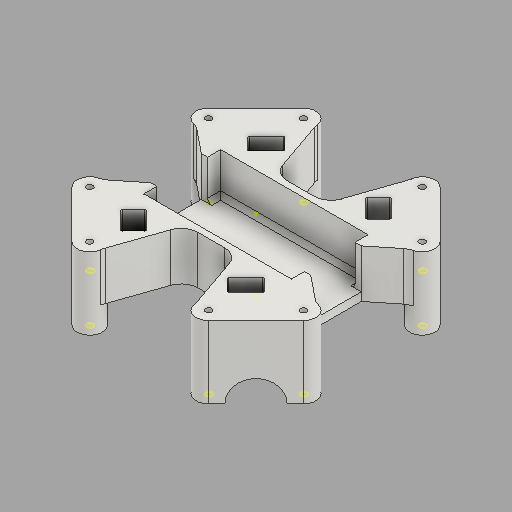
# Autodesk Inventor part: motor_converter
Saved by Autodesk Inventor 2023 (Build 270158000, 158)
## iProperties
Created: 2024-10-30
Part Number: motor_converter
Material: Полиэтилен, низкая плотность
Document SubType Name: Modeling
Designer: Ivan
Density: 0.894 g/cm^3
Appearance: Сталь
Mass: 114.342 g
Surface Area: 371.209 cm^2
Volume: 127.899 cm^3
Author: Ivan
Autodesk Inventor part; units mm, degrees
ref_plane "YZ Plane" through (0, 0, 0) normal (1, 0, 0) x (0, 1, 0)
ref_plane "XZ Plane" through (0, 0, 0) normal (0, 1, 0) x (-1, 0, 0)
ref_plane "XY Plane" through (0, 0, 0) normal (0, 0, 1) x (1, 0, 0)
derived "floor_v2.ipt"
sketch "Эскиз3" plane through (0, 2, 0) normal (0, -1, 0) x (-1, 0, 0)
  line L0 (33.8509, 77.6915) -> (77.6915, 33.8509) construction
  line L1 (55.7712, 55.7712) -> (0, 0) construction
  line L2 (44.4575, 67.0849) -> (67.0849, 44.4575) construction
  circle A0 centre (44.4575, 67.0849) radius 1.5
  circle A1 centre (67.0849, 44.4575) radius 1.5
  line L3 (28.3991, 51.0265) -> (51.0265, 28.3991) construction
  circle A2 centre (28.3991, 51.0265) radius 1.5
  circle A3 centre (51.0265, 28.3991) radius 1.5
  line L4 (44.4575, -67.0849) -> (67.0849, -44.4575) construction
  line L5 (28.3991, -51.0265) -> (51.0265, -28.3991) construction
  line L6 (55.7712, -55.7712) -> (0, 0) construction
  line L7 (-55.7712, -55.7712) -> (0, 0) construction
  line L8 (-28.3991, -51.0265) -> (-51.0265, -28.3991) construction
  line L9 (-44.4575, -67.0849) -> (-67.0849, -44.4575) construction
  line L10 (-55.7712, 55.7712) -> (0, 0) construction
  line L11 (-51.0265, 28.3991) -> (-28.3991, 51.0265) construction
  line L12 (-67.0849, 44.4575) -> (-44.4575, 67.0849) construction
  circle A4 centre (-44.4575, 67.0849) radius 1.5
  circle A5 centre (-67.0849, 44.4575) radius 1.5
  circle A6 centre (-28.3991, 51.0265) radius 1.5
  circle A7 centre (-51.0265, 28.3991) radius 1.5
  circle A8 centre (-44.4575, -67.0849) radius 1.5
  circle A9 centre (-67.0849, -44.4575) radius 1.5
  circle A10 centre (-51.0265, -28.3991) radius 1.5
  circle A11 centre (-28.3991, -51.0265) radius 1.5
  circle A12 centre (44.4575, -67.0849) radius 1.5
  circle A13 centre (28.3991, -51.0265) radius 1.5
  circle A14 centre (51.0265, -28.3991) radius 1.5
  circle A15 centre (67.0849, -44.4575) radius 1.5
  line L13 (-38.4471, -82.2877) -> (-82.2877, -38.4471)
  line L14 (82.2877, -38.4471) -> (38.4471, -82.2877)
  line L15 (38.4471, 82.2877) -> (82.2877, 38.4471)
  line L16 (-82.2877, 38.4471) -> (-38.4471, 82.2877)
  line L17 (82.2877, 38.4471) -> (92.1165, 48.2758)
  point P0 (39.7128, 39.7128)
  point P1 (-39.7128, -39.7128)
  point P2 (39.7128, -39.7128)
  point P3 (-39.7128, 39.7128)
  point P4 (-40.1306, -40.1306)
sketch "Эскиз6" plane through (0, 0, 0) normal (0, 1, 0) x (-1, 0, 0)
  circle A0 centre (28.3991, 51.0265) radius 1.5 projected
  circle A1 centre (51.0265, 28.3991) radius 1.5 projected
  line L0 (28.3991, -51.0265) -> (51.0265, -28.3991) construction
  circle A2 centre (28.3991, -51.0265) radius 1.5 projected
  circle A3 centre (-28.3991, -51.0265) radius 1.5 projected
  circle A4 centre (-51.0265, -28.3991) radius 1.5 projected
  circle A5 centre (-51.0265, 28.3991) radius 1.5 projected
  circle A6 centre (-28.3991, 51.0265) radius 1.5 projected
  circle A7 centre (51.0265, 28.3991) radius 6
  circle A8 centre (28.3991, 51.0265) radius 6
  circle A9 centre (51.0265, -28.3991) radius 6
  circle A10 centre (28.3991, -51.0265) radius 6
  circle A11 centre (-28.3991, -51.0265) radius 6
  circle A12 centre (-51.0265, -28.3991) radius 6
  circle A13 centre (-51.0265, 28.3991) radius 6
  circle A14 centre (-28.3991, 51.0265) radius 6
  line L1 (55.2691, 32.6417) -> (46.7838, 24.1564) construction
  line L2 (28.3991, 51.0265) -> (51.0265, 28.3991) construction
  line L3 (32.6417, 55.2691) -> (24.1564, 46.7838) construction
  line L4 (-28.3991, 51.0265) -> (-51.0265, 28.3991) construction
  line L5 (-51.0265, -28.3991) -> (-28.3991, -51.0265) construction
  line L6 (-32.6417, 55.2691) -> (-24.1564, 46.7838) construction
  line L7 (-55.2691, 32.6417) -> (-46.7838, 24.1564) construction
  line L8 (-46.7838, -24.1564) -> (-55.2691, -32.6417) construction
  line L9 (-24.1564, -46.7838) -> (-32.6417, -55.2691) construction
  line L10 (24.1564, -46.7838) -> (32.6417, -55.2691) construction
  line L11 (46.7838, -24.1564) -> (55.2691, -32.6417) construction
  line L12 (32.6417, 55.2691) -> (55.2691, 32.6417)
  line L13 (46.7838, 24.1564) -> (24.1564, 46.7838)
  line L14 (55.2691, -32.6417) -> (32.6417, -55.2691)
  line L15 (24.1564, -46.7838) -> (46.7838, -24.1564)
  line L16 (-24.1564, -46.7838) -> (-46.7838, -24.1564)
  line L17 (-55.2691, -32.6417) -> (-32.6417, -55.2691)
  line L18 (-24.1564, 46.7838) -> (-46.7838, 24.1564)
  line L19 (-55.2691, 32.6417) -> (-32.6417, 55.2691)
  circle A15 centre (51.0265, -28.3991) radius 1.5 projected
  point P0 (0, 0)
  point P1 (-32.6417, -55.2691)
  dimension "d19" = 12
  constraints: 32 end point, 16 point on circle, 15 coincident, 11 perpendicular, 8 midpoint, 7 centre point, 6 equal radius, 4 parallel, 3 tangent, 1 point on line, 4 other
  measures "d19" diameter of A7
extrude "Выдавливание2" add sketch "Эскиз6" against normal blind 34.5 contours A0 | A1 | A2 | A3 | A4 | A5 | A6 | A7 | A7 L13 A8 L12 | A8 | A9 | A9 L14 A10 L15 | A10 | A11 | A11 L17 A12 L16 | A12 | A13 | A13 L19 A14 L18 | A14 | A15
sketch "Эскиз7" plane through (32.6417, -34.5, 55.2691) normal (0.7071068, 0, 0.7071068) x (0.7071068, 0, -0.7071068)
  line L0 (32, 0) -> (0, 0) projected
  line L1 (32, 0) -> (0, 0) projected
  circle A0 centre (16, 0) radius 10.5
  point P0 (16, 34.5)
  point P1 (5.5, 0)
  point P2 (26.5, 0)
  dimension "d23" = 21
  constraints: 1 centre point, 1 midpoint
  measures "d23" diameter of A0
extrude "Выдавливание3" cut sketch "Эскиз7" against normal through all contours L0 A0 picked at (17.9882, 2.8804)
mirror "Зеркальное отражение1" about plane through (0, 0, 0) normal (0, 0, 1) of "Выдавливание3"
sketch "Эскиз8" plane through (0, 0, 0) normal (0, 1, 0) x (1, 0, 0)
  point P0 (0, 0)
sketch "Эскиз9" plane through (0, -34.5, 0) normal (0, -1, 0) x (1, 0, 0)
  circle A0 centre (-28.3991, 51.0265) radius 1.5 projected
  circle A1 centre (-51.0265, 28.3991) radius 1.5 projected
  circle A2 centre (28.3991, 51.0265) radius 1.5 projected
  circle A3 centre (51.0265, 28.3991) radius 1.5 projected
  circle A4 centre (51.0265, -28.3991) radius 1.5 projected
  circle A5 centre (28.3991, -51.0265) radius 1.5 projected
  circle A6 centre (-28.3991, -51.0265) radius 1.5 projected
  circle A7 centre (-51.0265, -28.3991) radius 1.5 projected
  point P0 (0, 0)
extrude "Выдавливание4" cut sketch "Эскиз3" along normal blind 9 contours A2 | A3 | A6 | A7 | A10 | A11 | A13 | A14
extrude "Выдавливание5" cut sketch "Эскиз9" against normal blind 7
sketch "Эскиз10" plane through (0, 0, 0) normal (0, 1, 0) x (1, 0, 0)
  line L0 (-35.225, -18.325) -> (-35.225, 18.325)
  line L1 (-35.225, 18.325) -> (35.225, 18.325)
  line L2 (35.225, 18.325) -> (35.225, -18.325)
  line L3 (35.225, -18.325) -> (-35.225, -18.325)
  circle A0 centre (-51.0265, 28.3991) radius 1.5 projected
  circle A1 centre (-51.0265, -28.3991) radius 1.5 projected
  circle A2 centre (-51.0265, 28.3991) radius 1.5 projected
  line L4 (-51.0265, 28.3991) -> (-51.0265, -28.3991) construction
  line L5 (-35.225, 18.325) -> (35.225, -18.325) construction
  line L6 (-38.225, 21.325) -> (38.225, 21.325)
  line L7 (38.225, 21.325) -> (38.225, -21.325)
  line L8 (38.225, -21.325) -> (-38.225, -21.325)
  line L9 (-38.225, -21.325) -> (-38.225, 21.325)
  line L10 (-38.225, 21.325) -> (38.225, -21.325) construction
  line L11 (-31, 15.1) -> (31, 15.1) construction
  line L12 (0, 0) -> (0, 15.1) construction
  circle A3 centre (-31, 15.1) radius 1.65
  circle A4 centre (31, 15.1) radius 1.65
  line L13 (-35.225, 0) -> (35.225, 0) construction
  circle A5 centre (-31, -15.1) radius 1.65
  circle A6 centre (31, -15.1) radius 1.65
  line L14 (-38.225, 12.1) -> (-35.225, 12.1)
  line L15 (-38.225, -12.1) -> (-35.225, -12.1)
  line L16 (38.225, 12.1) -> (35.225, 12.1)
  line L17 (38.225, -12.1) -> (35.225, -12.1)
  arc A7 (-24.1564, 46.7838) -> (-32.6417, 55.2691) centre (-28.3991, 51.0265) ccw projected
  arc A8 (-55.2691, 32.6417) -> (-46.7838, 24.1564) centre (-51.0265, 28.3991) ccw projected
  arc A9 (-46.7838, -24.1564) -> (-55.2691, -32.6417) centre (-51.0265, -28.3991) ccw projected
  arc A10 (-32.6417, -55.2691) -> (-24.1564, -46.7838) centre (-28.3991, -51.0265) ccw projected
  arc A11 (24.1564, -46.7838) -> (32.6417, -55.2691) centre (28.3991, -51.0265) ccw projected
  arc A12 (55.2691, -32.6417) -> (46.7838, -24.1564) centre (51.0265, -28.3991) ccw projected
  arc A13 (46.7838, 24.1564) -> (55.2691, 32.6417) centre (51.0265, 28.3991) ccw projected
  arc A14 (32.6417, 55.2691) -> (24.1564, 46.7838) centre (28.3991, 51.0265) ccw projected
  circle A15 centre (-28.3991, 51.0265) radius 1.5 projected
  line L18 (-28.3991, 51.0265) -> (-24.1564, 55.2691) construction
  line L19 (-28.3991, 51.0265) -> (-24.1564, 46.7838) construction
  arc A16 (-24.1564, 46.7838) -> (-32.6417, 55.2691) centre (-28.3991, 51.0265) ccw projected
  line L20 (-24.1564, 55.2691) -> (-24.1564, 46.7838) construction
  line L21 (-28.3991, 51.0265) -> (-22.3991, 51.0265)
  arc A17 (-22.3991, 51.0265) -> (0, 21.325) centre (3.3903, 47.1785) ccw
  arc A18 (-55.2691, 24.1564) -> (-38.225, 12.1) centre (-33.0894, 37.436) ccw
  line L22 (-46.7838, 24.1564) -> (-24.1564, 46.7838) projected
  point P0 (-24.1564, 51.0265)
  dimension "d31" = 70.45
  dimension "d32" = 36.65
  dimension "d33" = 76.45
  dimension "d34" = 42.65
  dimension "d35" = 3.225
  dimension "d36" = 4.225
  dimension "d37" = 3.3
  dimension "d38" = 3
  constraints: 44 end point, 8 point on circle, 8 symmetric about line, 7 midpoint, 6 centre point, 5 perpendicular, 4 parallel, 3 coincident, 3 point on line, 3 vertical, 2 horizontal, 1 equal radius, 2 other
  measures "d31" distance of L0.end L1.end
  measures "d32" distance of L1.end L2.end
  measures "d33" distance of L6.start L6.end
  measures "d34" distance of L6.end L7.end
  measures "d35" distance from line of L1 L12.end
  measures "d36" distance from line of L0 L11.start
  measures "d37" diameter of A3
  measures "d38" distance from line of L11 L14.end
extrude "Выдавливание6" add sketch "Эскиз10" against normal blind 17 contours L3 L2 L17 L7 L8 L9 L15 L0 | L14 L9 L6 L7 L16 L2 L1 L0
sketch "Эскиз11" plane through (0, -17, 0) normal (0, -1, 0) x (1, 0, 0)
  line L0 (-38.225, 21.325) -> (-38.225, 12.1) projected
  line L1 (-38.225, -21.325) -> (38.225, -21.325) projected
  line L2 (-38.225, 21.325) -> (38.225, 21.325)
  line L3 (38.225, 21.325) -> (38.225, -21.325)
  line L4 (38.225, -21.325) -> (-38.225, -21.325)
  line L5 (-38.225, -21.325) -> (-38.225, 21.325)
  circle A0 centre (-31, 15.1) radius 1.65 projected
  circle A1 centre (31, 15.1) radius 1.65 projected
  circle A2 centre (31, -15.1) radius 1.65 projected
  circle A3 centre (-31, -15.1) radius 1.65 projected
  point P0 (0, 0)
  constraints: 8 end point, 2 parallel, 1 horizontal, 1 perpendicular
extrude "Выдавливание7" add sketch "Эскиз11" along normal blind 5 contours L2 L3 L1 L5 L0 | A0 | A1 | A2 | A3
sketch "Эскиз12" plane through (0, 0, 0) normal (0, 1, 0) x (1, 0, 0)
  circle A0 centre (-51.0265, 28.3991) radius 1.5 projected
  circle A1 centre (-28.3991, 51.0265) radius 1.5 projected
  line L0 (-32.6417, 55.2691) -> (-55.2691, 32.6417) projected
  arc A2 (-55.2691, 32.6417) -> (-46.7838, 24.1564) centre (-51.0265, 28.3991) ccw projected
  line L1 (-46.7838, 24.1564) -> (-24.1564, 46.7838) projected
  arc A3 (-24.1564, 46.7838) -> (-32.6417, 55.2691) centre (-28.3991, 51.0265) ccw projected
  circle A4 centre (28.3991, 51.0265) radius 1.5 projected
  circle A5 centre (-28.3991, 51.0265) radius 1.5 projected
  line L2 (28.3991, 51.0265) -> (-28.3991, 51.0265) construction
  circle A6 centre (-51.0265, -28.3991) radius 1.5 projected
  line L3 (-51.0265, 28.3991) -> (-51.0265, -28.3991) construction
  arc A7 (-24.1564, 46.7838) -> (-32.6417, 55.2691) centre (-28.3991, 51.0265) ccw projected
  line L4 (38.225, 21.325) -> (-38.225, 21.325) projected
  line L5 (-38.225, 21.325) -> (-38.225, 12.1) projected
  arc A8 (-55.2691, 32.6417) -> (-46.7838, 24.1564) centre (-51.0265, 28.3991) ccw projected
  line L6 (-51.0265, 22.3991) -> (-38.225, 12.1)
  arc A9 (-24.1564, 46.7838) -> (-32.6417, 55.2691) centre (-28.3991, 51.0265) ccw projected
  line L7 (-22.3991, 51.0265) -> (-12.1, 21.325)
  arc A10 (32.6417, 55.2691) -> (24.1564, 46.7838) centre (28.3991, 51.0265) ccw projected
  line L8 (22.3991, 51.0265) -> (12.1, 21.325)
  arc A11 (46.7838, 24.1564) -> (55.2691, 32.6417) centre (51.0265, 28.3991) ccw projected
  circle A12 centre (51.0265, -28.3991) radius 1.5 projected
  line L9 (51.0265, 28.3991) -> (51.0265, -28.3991) construction
  circle A13 centre (28.3991, -51.0265) radius 1.5 projected
  circle A14 centre (-28.3991, -51.0265) radius 1.5 projected
  line L10 (28.3991, -51.0265) -> (-28.3991, -51.0265) construction
  line L11 (35.225, 12.1) -> (38.225, 12.1) projected
  line L12 (38.225, 12.1) -> (51.0265, 22.3991)
  line L13 (38.225, 12.1) -> (38.225, -12.1) projected
  line L14 (38.225, -12.1) -> (51.0265, -22.3991)
  arc A15 (55.2691, -32.6417) -> (46.7838, -24.1564) centre (51.0265, -28.3991) ccw projected
  arc A16 (24.1564, -46.7838) -> (32.6417, -55.2691) centre (28.3991, -51.0265) ccw projected
  line L15 (22.3991, -51.0265) -> (12.1, -21.325)
  line L16 (38.225, -21.325) -> (-38.225, -21.325) projected
  arc A17 (-32.6417, -55.2691) -> (-24.1564, -46.7838) centre (-28.3991, -51.0265) ccw projected
  line L17 (-38.225, -21.325) -> (38.225, -21.325) projected
  line L18 (-22.3991, -51.0265) -> (-12.1, -21.325)
  line L19 (-38.225, -12.1) -> (-38.225, -21.325) projected
  line L20 (-38.225, -12.1) -> (-51.0265, -22.3991)
  arc A18 (-46.7838, -24.1564) -> (-55.2691, -32.6417) centre (-51.0265, -28.3991) ccw projected
  circle A19 centre (28.3991, 51.0265) radius 1.5 projected
  circle A20 centre (51.0265, 28.3991) radius 1.5 projected
  arc A21 (46.7838, 24.1564) -> (55.2691, 32.6417) centre (51.0265, 28.3991) ccw projected
  line L21 (55.2691, 32.6417) -> (32.6417, 55.2691) projected
  arc A22 (32.6417, 55.2691) -> (24.1564, 46.7838) centre (28.3991, 51.0265) ccw projected
  line L22 (24.1564, 46.7838) -> (46.7838, 24.1564) projected
  circle A23 centre (28.3991, -51.0265) radius 1.5 projected
  circle A24 centre (51.0265, -28.3991) radius 1.5 projected
  line L23 (46.7838, -24.1564) -> (24.1564, -46.7838) projected
  arc A25 (24.1564, -46.7838) -> (32.6417, -55.2691) centre (28.3991, -51.0265) ccw projected
  line L24 (32.6417, -55.2691) -> (55.2691, -32.6417) projected
  arc A26 (55.2691, -32.6417) -> (46.7838, -24.1564) centre (51.0265, -28.3991) ccw projected
  circle A27 centre (-28.3991, -51.0265) radius 1.5 projected
  circle A28 centre (-51.0265, -28.3991) radius 1.5 projected
  line L25 (-24.1564, -46.7838) -> (-46.7838, -24.1564) projected
  arc A29 (-46.7838, -24.1564) -> (-55.2691, -32.6417) centre (-51.0265, -28.3991) ccw projected
  line L26 (-55.2691, -32.6417) -> (-32.6417, -55.2691) projected
  arc A30 (-32.6417, -55.2691) -> (-24.1564, -46.7838) centre (-28.3991, -51.0265) ccw projected
  line L27 (38.225, 12.1) -> (38.225, 21.325) projected
  line L28 (38.225, -21.325) -> (38.225, -12.1) projected
  line L29 (-19.3804, 33.1638) -> (-25.3908, 39.1742)
  line L30 (-25.3908, 39.1742) -> (-34.2296, 30.3354)
  line L31 (-34.2296, 30.3354) -> (-28.2192, 24.325)
  line L32 (-28.2192, 24.325) -> (-19.3804, 33.1638)
  line L33 (0, 51.0265) -> (0, -51.0265) construction
  line L34 (19.3804, 33.1638) -> (25.3908, 39.1742)
  line L35 (25.3908, 39.1742) -> (34.2296, 30.3354)
  line L36 (34.2296, 30.3354) -> (28.2192, 24.325)
  line L37 (28.2192, 24.325) -> (19.3804, 33.1638)
  line L38 (51.0265, 0) -> (-51.0265, 0) construction
  line L39 (-19.3804, -33.1638) -> (-25.3908, -39.1742)
  line L40 (-25.3908, -39.1742) -> (-34.2296, -30.3354)
  line L41 (-34.2296, -30.3354) -> (-28.2192, -24.325)
  line L42 (-28.2192, -24.325) -> (-19.3804, -33.1638)
  line L43 (28.2192, -24.325) -> (19.3804, -33.1638)
  line L44 (19.3804, -33.1638) -> (25.3908, -39.1742)
  line L45 (25.3908, -39.1742) -> (34.2296, -30.3354)
  line L46 (34.2296, -30.3354) -> (28.2192, -24.325)
  point P0 (0, 0)
  point P1 (0, 21.325)
  point P2 (-46.7838, -24.1564)
  point P3 (-24.1564, -46.7838)
  point P4 (46.7838, 24.1564)
  point P5 (24.1564, 46.7838)
  point P6 (46.7838, -24.1564)
  dimension "d47" = 12.1
  dimension "d50" = 3
  dimension "d51" = 3
  dimension "d52" = 8.5
  dimension "d53" = 12.5
  constraints: 60 end point, 12 point on line, 12 symmetric about line, 8 point on circle, 5 midpoint, 3 equal length, 3 parallel, 3 vertical, 2 horizontal, 1 perpendicular
  measures "d47" distance of L7.end point (0, 21.325)
  measures "d50" distance from line of L4 L31.end
  measures "d51" distance from line of L7 L29.start
  measures "d52" distance from line of L32 L29.end
  measures "d53" distance from line of L31 L29.end
extrude "Выдавливание10" add sketch "Эскиз12" against normal up to surface (22 mm away) contours L7 L4 L5 L6 A2 L1 A3 | L4 L8 A10 L22 A11 L12 L27 | L14 A15 L23 A16 L15 L16 L28 | L18 A17 L25 A18 L20 L19 L16
fillet "Сопряжение1" radius 0.5 16 edges at (34.2296, -11, -30.3354) (28.2192, -11, -24.325) (19.3804, -11, -33.1638) (25.3908, -11, -39.1742) (-34.2296, -11, -30.3354) (-28.2192, -11, -24.325) (-19.3804, -11, -33.1638) (-25.3908, -11, -39.1742) (-25.3908, -11, 39.1742) (-19.3804, -11, 33.1638) (-34.2296, -11, 30.3354) (-28.2192, -11, 24.325) (25.3908, -11, 39.1742) (34.2296, -11, 30.3354) (19.3804, -11, 33.1638) (28.2192, -11, 24.325)
fillet "Сопряжение2" radius 8 12 edges at (22.3991, -11, -51.0265) (51.0265, -11, -22.3991) (51.0265, -11, 22.3991) (22.3991, -11, 51.0265) (-51.0265, -11, 22.3991) (-22.3991, -11, 51.0265) (-51.0265, -11, -22.3991) (-22.3991, -11, -51.0265) (12.1, -11, 21.325) (-12.1, -11, 21.325) (12.1, -11, -21.325) (-12.1, -11, -21.325)
sketch "Эскиз13" plane through (0, -22, 0) normal (0, -1, 0) x (1, 0, 0)
  line L0 (-33.8761, 29.9819) -> (-28.5728, 24.6786) projected
  arc A0 (-33.8761, 30.689) -> (-33.8761, 29.9819) centre (-33.5225, 30.3354) ccw projected
  line L1 (-25.7443, 38.8207) -> (-33.8761, 30.689) projected
  arc A1 (-25.0372, 38.8207) -> (-25.7443, 38.8207) centre (-25.3908, 38.4671) ccw projected
  line L2 (-19.7339, 33.5174) -> (-25.0372, 38.8207) projected
  arc A2 (-19.7339, 32.8103) -> (-19.7339, 33.5174) centre (-20.0875, 33.1638) ccw projected
  line L3 (-27.8657, 24.6786) -> (-19.7339, 32.8103) projected
  arc A3 (-28.5728, 24.6786) -> (-27.8657, 24.6786) centre (-28.2192, 25.0321) ccw projected
  line L4 (19.7339, -33.5174) -> (25.0372, -38.8207) projected
  arc A4 (19.7339, -32.8103) -> (19.7339, -33.5174) centre (20.0875, -33.1638) ccw projected
  line L5 (27.8657, -24.6786) -> (19.7339, -32.8103) projected
  arc A5 (28.5728, -24.6786) -> (27.8657, -24.6786) centre (28.2192, -25.0321) ccw projected
  line L6 (33.8761, -29.9819) -> (28.5728, -24.6786) projected
  arc A6 (33.8761, -30.689) -> (33.8761, -29.9819) centre (33.5225, -30.3354) ccw projected
  line L7 (25.7443, -38.8207) -> (33.8761, -30.689) projected
  arc A7 (25.0372, -38.8207) -> (25.7443, -38.8207) centre (25.3908, -38.4671) ccw projected
  line L8 (-33.8761, -30.689) -> (-25.7443, -38.8207) projected
  arc A8 (-33.8761, -29.9819) -> (-33.8761, -30.689) centre (-33.5225, -30.3354) ccw projected
  line L9 (-28.5728, -24.6786) -> (-33.8761, -29.9819) projected
  arc A9 (-27.8657, -24.6786) -> (-28.5728, -24.6786) centre (-28.2192, -25.0321) ccw projected
  line L10 (-19.7339, -32.8103) -> (-27.8657, -24.6786) projected
  arc A10 (-19.7339, -33.5174) -> (-19.7339, -32.8103) centre (-20.0875, -33.1638) ccw projected
  line L11 (-25.0372, -38.8207) -> (-19.7339, -33.5174) projected
  arc A11 (-25.7443, -38.8207) -> (-25.0372, -38.8207) centre (-25.3908, -38.4671) ccw projected
  line L12 (25.0372, 38.8207) -> (19.7339, 33.5174) projected
  arc A12 (25.7443, 38.8207) -> (25.0372, 38.8207) centre (25.3908, 38.4671) ccw projected
  line L13 (33.8761, 30.689) -> (25.7443, 38.8207) projected
  arc A13 (33.8761, 29.9819) -> (33.8761, 30.689) centre (33.5225, 30.3354) ccw projected
  line L14 (28.5728, 24.6786) -> (33.8761, 29.9819) projected
  arc A14 (27.8657, 24.6786) -> (28.5728, 24.6786) centre (28.2192, 25.0321) ccw projected
  line L15 (19.7339, 32.8103) -> (27.8657, 24.6786) projected
  arc A15 (19.7339, 33.5174) -> (19.7339, 32.8103) centre (20.0875, 33.1638) ccw projected
  line L16 (-38.225, 12.1) -> (-38.225, -12.1) projected
  line L17 (-49.3246, -21.0299) -> (-38.225, -12.1) projected
  arc A16 (-52.4463, -22.5695) -> (-49.3246, -21.0299) centre (-54.3393, -14.7967) ccw projected
  arc A17 (-46.7838, -24.1564) -> (-52.4463, -22.5695) centre (-51.0265, -28.3991) ccw projected
  line L18 (-24.1564, -46.7838) -> (-46.7838, -24.1564) projected
  arc A18 (-22.4393, -51.72) -> (-24.1564, -46.7838) centre (-28.3991, -51.0265) ccw projected
  arc A19 (-22.0514, -50.0239) -> (-22.4393, -51.72) centre (-14.4929, -52.6448) ccw projected
  line L19 (-13.9652, -26.7041) -> (-22.0514, -50.0239) projected
  arc A20 (-6.4067, -21.325) -> (-13.9652, -26.7041) centre (-6.4067, -29.325) ccw projected
  line L20 (-6.4067, -21.325) -> (6.4067, -21.325) projected
  arc A21 (13.9652, -26.7041) -> (6.4067, -21.325) centre (6.4067, -29.325) ccw projected
  line L21 (22.0514, -50.0239) -> (13.9652, -26.7041) projected
  arc A22 (22.4393, -51.72) -> (22.0514, -50.0239) centre (14.4929, -52.6448) ccw projected
  arc A23 (24.1564, -46.7838) -> (22.4393, -51.72) centre (28.3991, -51.0265) ccw projected
  line L22 (46.7838, -24.1564) -> (24.1564, -46.7838) projected
  arc A24 (52.4463, -22.5695) -> (46.7838, -24.1564) centre (51.0265, -28.3991) ccw projected
  arc A25 (49.3246, -21.0299) -> (52.4463, -22.5695) centre (54.3393, -14.7967) ccw projected
  line L23 (38.225, -12.1) -> (49.3246, -21.0299) projected
  line L24 (38.225, -12.1) -> (38.225, 12.1) projected
  line L25 (49.3246, 21.0299) -> (38.225, 12.1) projected
  arc A26 (52.4463, 22.5695) -> (49.3246, 21.0299) centre (54.3393, 14.7967) ccw projected
  arc A27 (46.7838, 24.1564) -> (52.4463, 22.5695) centre (51.0265, 28.3991) ccw projected
  line L26 (24.1564, 46.7838) -> (46.7838, 24.1564) projected
  arc A28 (22.4393, 51.72) -> (24.1564, 46.7838) centre (28.3991, 51.0265) ccw projected
  arc A29 (22.0514, 50.0239) -> (22.4393, 51.72) centre (14.4929, 52.6448) ccw projected
  line L27 (13.9652, 26.7041) -> (22.0514, 50.0239) projected
  arc A30 (6.4067, 21.325) -> (13.9652, 26.7041) centre (6.4067, 29.325) ccw projected
  line L28 (6.4067, 21.325) -> (-6.4067, 21.325) projected
  arc A31 (-13.9652, 26.7041) -> (-6.4067, 21.325) centre (-6.4067, 29.325) ccw projected
  line L29 (-22.0514, 50.0239) -> (-13.9652, 26.7041) projected
  arc A32 (-22.4393, 51.72) -> (-22.0514, 50.0239) centre (-14.4929, 52.6448) ccw projected
  arc A33 (-24.1564, 46.7838) -> (-22.4393, 51.72) centre (-28.3991, 51.0265) ccw projected
  line L30 (-46.7838, 24.1564) -> (-24.1564, 46.7838) projected
  arc A34 (-52.4463, 22.5695) -> (-46.7838, 24.1564) centre (-51.0265, 28.3991) ccw projected
  arc A35 (-49.3246, 21.0299) -> (-52.4463, 22.5695) centre (-54.3393, 14.7967) ccw projected
  line L31 (-38.225, 12.1) -> (-49.3246, 21.0299) projected
  point P0 (0, 0)
extrude "Выдавливание11" add sketch "Эскиз13" along normal blind 1
sketch "Эскиз14" plane through (0, -17, 0) normal (0, 1, 0) x (1, 0, 0)
  line L0 (-35.225, 12.1) -> (-38.225, 12.1) projected
  line L1 (-38.225, -12.1) -> (-38.225, 12.1) projected
  line L2 (-38.225, -12.1) -> (-35.225, -12.1) projected
  line L3 (-35.225, -12.1) -> (-35.225, -18.325) projected
  line L4 (-35.225, -18.325) -> (35.225, -18.325) projected
  line L5 (35.225, -18.325) -> (35.225, -12.1) projected
  line L6 (35.225, -12.1) -> (38.225, -12.1) projected
  line L7 (38.225, 12.1) -> (38.225, -12.1) projected
  line L8 (38.225, 12.1) -> (35.225, 12.1) projected
  line L9 (35.225, 12.1) -> (35.225, 18.325) projected
  line L10 (35.225, 18.325) -> (-35.225, 18.325) projected
  line L11 (-35.225, 18.325) -> (-35.225, 12.1) projected
  point P0 (0, 0)
extrude "Выдавливание12" cut sketch "Эскиз14" against normal blind 2
fillet "Сопряжение3" radius 2 6 edges at (0, -19, -18.325) (-35.225, -19, -15.2125) (35.225, -19, -15.2125) (35.225, -19, 15.2125) (0, -19, 18.325) (-35.225, -19, 15.2125)
